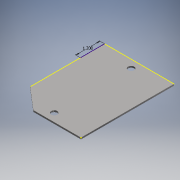
# Autodesk Inventor part: Flywheel Motor Plate
Saved by Autodesk Inventor 2017 (Build 210142000, 142)
## iProperties
Created: 2016-10-11
Part Number: Flywheel Motor Plate
Material: Steel, Alloy
Document SubType Name: Modeling
Designer: Aditya
Density: 7.73 g/cm^3
Appearance: Semi-Polished
Author: Aditya
Autodesk Inventor part; units mm, degrees
ref_plane "YZ Plane" through (0, 0, 0) normal (1, 0, 0) x (0, 1, 0)
ref_plane "XZ Plane" through (0, 0, 0) normal (0, 1, 0) x (-1, 0, 0)
ref_plane "XY Plane" through (0, 0, 0) normal (0, 0, 1) x (1, 0, 0)
sketch "Sketch1" plane through (0, 0, 0) normal (0, 1, 0) x (-1, 0, 0)
  line L0 (0, 0) -> (0, -117.094)
  line L1 (0, -117.094) -> (87.63, -117.094)
  line L2 (87.63, -117.094) -> (87.63, -23.622)
  line L3 (0, 0) -> (59.944, 0)
  line L4 (59.944, 0) -> (87.63, -23.622)
  circle A0 centre (43.815, -106.934) radius 3.937
  circle A1 centre (43.815, -10.16) radius 3.937
  line L5 (87.63, -117.094) -> (80.01, -117.094)
  dimension "d0" = 117.094
  dimension "d1" = 87.63
  dimension "d2" = 93.472
  dimension "d3" = 59.944
  dimension "d10" = 7.62
  constraints: 12 end point, 2 centre point, 2 perpendicular, 1 horizontal, 1 point on line, 1 vertical
  measures "d0" distance of L0.start L0.end
  measures "d1" distance of L0.end L1.end
  measures "d2" distance of L1.end L2.end
  measures "d3" distance of L0.start L3.end
  measures "d10" distance of L1.end L5.end
extrude "Extrusion3" add sketch "Sketch1" along normal blind 1.9558
sketch "Sketch2" plane through (0, 1.9558, 0) normal (0, 1, 0) x (1, 0, 0)
  line L0 (0, 117.094) -> (-87.63, 117.094) projected
  line L1 (-87.63, 117.094) -> (-87.63, 86.614)
  line L2 (-87.63, 117.094) -> (-87.63, 23.622) projected
  point P0 (0, 0)
  dimension "d19" = 30.48
  constraints: 2 end point, 1 point on line
  measures "d19" distance of L0.end L1.end
sketch "Sketch3" plane through (0, 1.9558, 0) normal (0, 1, 0) x (1, 0, 0)
  line L0 (-83.82, 52.774) -> (-83.82, 84.1388) projected
  line L1 (-76.2, 52.774) -> (-83.82, 52.774) projected
  line L2 (-76.2, 84.1388) -> (-76.2, 52.774) projected
  line L3 (-76.2, 84.1388) -> (-83.82, 84.1388) projected
  circle A0 centre (-80.01, 58.9314) radius 2.0193 projected
  circle A1 centre (-80.01, 77.9814) radius 2.0193 projected
  point P0 (0, 0)
extrude "Extrusion4" cut sketch "Sketch3" against normal blind 25.4 contours A0 | A1
body "Solid3"
